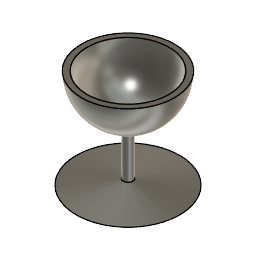
EX-4.2 (Autodesk Fusion 360 design; units mm, degrees)
part number: 2026-05-09-13-46-18-352
Autodesk Fusion 360 part; units mm, degrees
sketch "Sketch1" plane through (0, 0, 0) normal (0, 1, 0) x (1, 0, 0)
  line L0 (0, 0) -> (0, -1.501)
  line L1 (-1.0574, -2.5575) -> (-1.2054, -2.5575)
  line L2 (0, 0) -> (-1.336, 0)
  line L3 (-1.336, 0) -> (-0.123, -0.148)
  line L4 (-0.123, -0.148) -> (-0.123, -1.3618)
  arc A0 (0, -1.501) -> (-1.0574, -2.5575) centre (-0.0009, -2.5575) ccw
  arc A1 (-0.123, -1.3618) -> (-1.2028, -2.5575) centre (-0.0009, -2.5575) ccw
  line L5 (0, 0) -> (0, -3.8)
  dimension "d1" = 1.501
  dimension "d2" = 2.113
  dimension "d3" = 0.148
  dimension "d4" = 1.336
  dimension "d5" = 0.123
  dimension "d6" = 0.148
  constraint coincident L0.start L2.start
  constraint vertical L0
  constraint horizontal L1
  constraint concentric A0 A1
  constraint perpendicular L0 L2
  constraint perpendicular L2 L4
  constraint coincident L1 A1.end
  measures "d1" distance of L0.start L0.end
  measures "d2" diameter of A0
  measures "d3" distance of L1.start L1.end
  measures "d4" distance of L0.start L2.end
  measures "d5" distance of L0 L4
  measures "d6" distance of L2 L3.end
revolve "Revolve1" add sketch "Sketch1" angle 360 about axis through (0, 0, 0) along (0, 0, 1)
